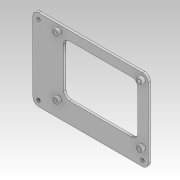
# Autodesk Inventor part: NewMoboAdapter
Saved by Autodesk Inventor 2020 (Build 240168000, 168)
## iProperties
Created: 2022-08-31
Part Number: NewMoboAdapter
Material: Generic
Document SubType Name: Modeling
Designer: DDeGo
Density: 1 g/cm^3
Appearance: Default
Author: DDeGo
Autodesk Inventor part; units mm, degrees
ref_plane "YZ Plane" through (0, 0, 0) normal (1, 0, 0) x (0, 1, 0)
ref_plane "XZ Plane" through (0, 0, 0) normal (0, 1, 0) x (-1, 0, 0)
ref_plane "XY Plane" through (0, 0, 0) normal (0, 0, 1) x (1, 0, 0)
sketch "Sketch1" plane through (0, 0, 0) normal (0, 0, 1) x (1, 0, 0)
  line L0 (-37.05, 26) -> (37.05, 26) construction
  line L1 (37.05, 26) -> (37.05, -26) construction
  line L2 (37.05, -26) -> (-37.05, -26) construction
  line L3 (-37.05, -26) -> (-37.05, 26) construction
  line L4 (-37.05, 26) -> (37.05, -26) construction
  line L5 (37.05, 26) -> (-37.05, -26) construction
  circle A0 centre (37.05, 26) radius 1.5
  circle A1 centre (37.05, -26) radius 1.5
  circle A2 centre (-37.05, -26) radius 1.5
  circle A3 centre (-37.05, 26) radius 1.5
  line L6 (0, 45) -> (0, 0) construction
  line L7 (-18.2065, -55) -> (-18.2065, -15) construction
  circle A4 centre (37.05, 26) radius 3 construction
  circle A5 centre (37.05, -26) radius 3 construction
  circle A6 centre (-37.05, -26) radius 3 construction
  circle A7 centre (-37.05, 26) radius 3 construction
  line L8 (37.05, 26) -> (-54.95, 26) construction
  line L9 (-54.95, 26) -> (-54.95, -36) construction
  line L10 (-54.95, -36) -> (37.05, -36) construction
  line L11 (37.05, -36) -> (37.05, 26) construction
  circle A8 centre (-54.95, 26) radius 1.5
  circle A9 centre (-54.95, -36) radius 1.5
  circle A10 centre (37.05, -36) radius 1.5
  line L12 (-54.95, 31) -> (37.05, 31)
  line L13 (42.05, 26) -> (42.05, -36)
  line L14 (37.05, -41) -> (-54.95, -41)
  line L15 (-59.95, -36) -> (-59.95, 26)
  arc A11 (-54.95, 31) -> (-59.95, 26) centre (-54.95, 26) ccw
  arc A12 (-59.95, -36) -> (-54.95, -41) centre (-54.95, -36) ccw
  arc A13 (37.05, -41) -> (42.05, -36) centre (37.05, -36) ccw
  arc A14 (42.05, 26) -> (37.05, 31) centre (37.05, 26) ccw
  line L16 (27.775, -23) -> (-27.775, -23)
  line L17 (-32.775, -18) -> (-32.775, 18)
  line L18 (-27.775, 23) -> (27.775, 23)
  line L19 (32.775, 18) -> (32.775, -18)
  line L20 (32.775, -23) -> (-32.775, 23) construction
  line L21 (-32.775, -23) -> (32.775, 23) construction
  arc A15 (-27.775, 23) -> (-32.775, 18) centre (-27.775, 18) ccw
  arc A16 (32.775, 18) -> (27.775, 23) centre (27.775, 18) ccw
  arc A17 (27.775, -23) -> (32.775, -18) centre (27.775, -18) ccw
  arc A18 (-32.775, -18) -> (-27.775, -23) centre (-27.775, -18) ccw
  point P0 (0, 0)
  point P1 (0, 0)
  dimension "d0" = 74.1
  dimension "d1" = 52
  dimension "d2" = 3
  dimension "d3" = 45
  dimension "d4" = 6
  dimension "d5" = 0
  dimension "d8" = 62
  dimension "d9" = 92
  dimension "d10" = 5
  dimension "d11" = 5
  dimension "d12" = 5
  dimension "d13" = 5
  dimension "d14" = 5
  dimension "d15" = 5
  dimension "d16" = 3
  constraints: 44 end point, 19 centre point, 16 point on circle, 16 tangent, 15 equal radius, 13 coincident, 9 parallel, 9 point on line, 4 horizontal, 4 perpendicular, 3 midpoint, 2 other
  measures "d0" distance of L2.start L5.end
  measures "d1" distance of L5.start L2.start
  measures "d2" diameter of A1
  measures "d3" distance of L6.start L6.end
  measures "d4" diameter of A4
  measures "d5" distance of L6.end point (0, 0)
  measures "d8" distance of L10.end L8.start
  measures "d9" distance of L9.end L10.end
  measures "d10" distance between parallel lines of L13 L1
  measures "d11" distance between parallel lines of L0 L12
  measures "d12" distance between parallel lines of L15 L9
  measures "d13" distance between parallel lines of L14 L10
  measures "d14" radius of A11
  measures "d15" radius of A15
  measures "d16" distance between parallel lines of L8 L18
extrude "Extrusion1" add sketch "Sketch1" along normal blind 2
sketch "Sketch2" plane through (0, 0, 2) normal (0, 0, 1) x (1, 0, 0)
  circle A0 centre (-37.05, 26) radius 1.5 projected
  circle A1 centre (-37.05, 26) radius 2.5
  circle A2 centre (37.05, 26) radius 1.5 projected
  circle A3 centre (37.05, 26) radius 2.5
  circle A4 centre (37.05, -26) radius 1.5 projected
  circle A5 centre (37.05, -26) radius 2.5
  circle A6 centre (-37.05, -26) radius 1.5 projected
  circle A7 centre (-37.05, -26) radius 2.5
  point P0 (0, 0)
  dimension "d19" = 5
  constraints: 4 centre point, 4 coincident, 3 equal radius
  measures "d19" diameter of A1
extrude "Extrusion2" add sketch "Sketch2" along normal blind 3
body "Solid1"
